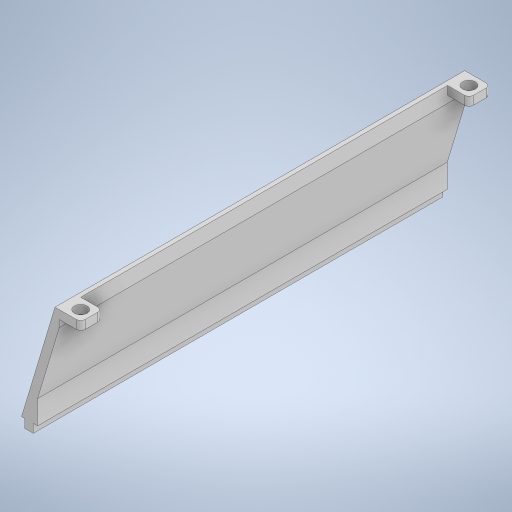
# Autodesk Inventor part: Přední rampa POKUS
Saved by Autodesk Inventor 2024 (Build 280153000, 153)
## iProperties
Created: 2023-05-12
Part Number: Přední rampa POKUS
Material: Všeobecné
Document SubType Name: Modeling
Designer: jaryj
Density: 1 g/cm^3
Appearance: Výchozí
Author: jaryj
Autodesk Inventor part; units mm, degrees
ref_plane "YZ Plane" through (0, 0, 0) normal (1, 0, 0) x (0, 1, 0)
ref_plane "XZ Plane" through (0, 0, 0) normal (0, 1, 0) x (-1, 0, 0)
ref_plane "XY Plane" through (0, 0, 0) normal (0, 0, 1) x (1, 0, 0)
sketch "Náčrt1" plane through (0, 0, 0) normal (0, 0, 1) x (1, 0, 0)
  line L0 (0, 0) -> (7.8004, 26)
  line L1 (0, 0) -> (0.7381, 0)
  line L2 (0.7381, 0) -> (0.7381, -2)
  line L3 (0.7381, -2) -> (2.7381, -2)
  line L4 (2.7381, -2) -> (2.7381, 0)
  line L5 (2.7381, 0) -> (3.7381, 0)
  line L6 (3.7381, 0) -> (3.7381, 5.5)
  line L7 (3.7381, 5.5) -> (8.8004, 22.3733)
  line L8 (8.8004, 22.3733) -> (8.8004, 26)
  line L9 (8.8004, 26) -> (7.8004, 26)
  line L10 (3.7381, 0) -> (18.7381, 0) construction
  dimension "d0" = 2
  dimension "d1" = 2
  dimension "d2" = 1
  dimension "d4" = 5.5
  dimension "d5" = 2
  dimension "d6" = 1
  dimension "d7" = 26
  dimension "d9" = 73.3
  dimension "d10" = 15
  constraints: 22 end point, 5 perpendicular, 2 horizontal, 2 point on line, 1 parallel, 1 vertical
  measures "d0" distance of L2.end L3.end
  measures "d1" distance of L3.end L4.end
  measures "d2" distance of L4.end L5.end
  measures "d4" distance of L5.end L6.end
  measures "d5" distance between parallel lines of L0 L7
  measures "d6" distance of L8.end L0.end
  measures "d7" distance between parallel lines of L5 L9
  measures "d9" angle of L7 L10
  measures "d10" distance of L5.end L10.end
extrude "Vysunutí1" add sketch "Náčrt1" along normal blind 47.75
sketch "Náčrt2" plane through (7.8004, 26, 0) normal (0, 1, 0) x (1, 0, 0)
  line L0 (1, 0) -> (1, -47.75) projected
  line L1 (1, 0) -> (6, 0)
  line L2 (6, 0) -> (6, -5)
  line L3 (6, -5) -> (1, -5)
  line L4 (1, -5) -> (1, 0)
  point P0 (-7.8004, 0)
  point P1 (1, -5)
  dimension "d13" = 5
  dimension "d14" = 5
  constraints: 8 end point, 2 parallel, 1 horizontal, 1 perpendicular
  measures "d13" distance of L2.end L3.end
  measures "d14" distance of L1.end L2.end
extrude "Vysunutí2" add sketch "Náčrt2" against normal blind 2
sketch "Náčrt3" plane through (7.8004, 26, 47.75) normal (0, 1, 0) x (1, 0, 0)
  line L0 (1, 42.75) -> (6, 42.75) projected
  line L1 (6, 42.75) -> (6, 47.75) projected
  point P0 (-7.8004, 47.75)
  point P1 (3.5, 45.25)
  dimension "d17" = 2.5
  dimension "d25" = 2.5
  measures "d17" distance from line of L0 point (3.5, 45.25)
  measures "d25" distance from line of L1 point (3.5, 45.25)
hole "Díra1" at (11.3004, 26, 2.5) direction (0, -1, 0) diameter 3 depth 6
fillet "Zaoblení1" radius 1 2 edges at (13.8004, 25, 5) (13.8004, 25, 0)
mirror "Zrcadlit1" about plane through (4.4002, 12, 47.75) normal (0, 0, 1)
